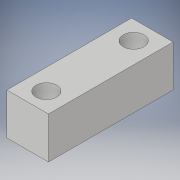
# Autodesk Inventor part: BaseBancada
Saved by Autodesk Inventor 2019 (Build 230136000, 136)
## iProperties
Created: 2019-07-02
Part Number: BaseBancada
Material: Generic
Document SubType Name: Modeling
Designer: Oscar Rojas
Density: 1 g/cm^3
Appearance: Default
Author: Oscar Rojas
Autodesk Inventor part; units mm, degrees
ref_plane "YZ Plane" through (0, 0, 0) normal (1, 0, 0) x (0, 1, 0)
ref_plane "XZ Plane" through (0, 0, 0) normal (0, 1, 0) x (-1, 0, 0)
ref_plane "XY Plane" through (0, 0, 0) normal (0, 0, 1) x (1, 0, 0)
sketch "Sketch1" plane through (0, 0, 0) normal (0, 1, 0) x (-1, 0, 0)
  line L0 (0, 0) -> (-20, 0)
  line L1 (-20, 0) -> (-20, -60)
  line L2 (-20, -60) -> (0, -60)
  line L3 (0, -60) -> (0, 0)
  dimension "d0" = 20
  dimension "d1" = 60
  constraints: 8 end point, 2 parallel, 1 horizontal, 1 perpendicular
  measures "d0" distance of L2.end L1.end
  measures "d1" distance of L1.end L0.end
extrude "Extrusion1" add sketch "Sketch1" along normal blind 20
sketch "Sketch2" plane through (0, 20, 0) normal (0, 1, 0) x (1, 0, 0)
  line L0 (0, 0) -> (20, 0) projected
  line L1 (10, 0) -> (10, 9)
  line L2 (10, 0) -> (19, 0) construction
  circle A0 centre (10, 9) radius 5
  line L3 (20, 60) -> (0, 60) projected
  line L4 (0, 0) -> (0, 60)
  line L5 (0, 60) -> (0, 0) projected
  line L6 (0, 30) -> (2.0385, 30)
  circle A1 centre (10, 51) radius 5
  dimension "d5" = 9
  dimension "d6" = 90
  dimension "d7" = 10
  constraints: 8 end point, 2 centre point, 2 horizontal, 2 midpoint, 2 vertical, 1 coincident, 1 perpendicular, 1 symmetric about line, 1 other
  measures "d5" distance of L1.start L1.end
  measures "d6" angle of L2 L1
  measures "d7" diameter of A0
extrude "Extrusion2" cut sketch "Sketch2" against normal blind 23
body "Solid1"
